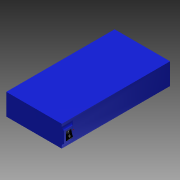
# Autodesk Inventor part: 12 Volt Battery Pack
Saved by Autodesk Inventor 2014 (Build 180170000, 170)
## iProperties
Created: 2014-02-26
Part Number: 12 Volt Battery Pack
Material: Generic
Document SubType Name: Modeling
Designer: Spooner
Density: 1 g/cm^3
Appearance: Blue - Wall Paint - Glossy
Author: Spooner
Autodesk Inventor part; units mm, degrees
ref_plane "YZ Plane" through (0, 0, 0) normal (1, 0, 0) x (0, 1, 0)
ref_plane "XZ Plane" through (0, 0, 0) normal (0, 1, 0) x (-1, 0, 0)
ref_plane "XY Plane" through (0, 0, 0) normal (0, 0, 1) x (1, 0, 0)
sketch "Sketch1" plane through (0, 0, 0) normal (0, 1, 0) x (-1, 0, 0)
  line L0 (0, 0) -> (-65.786, 0)
  line L1 (-65.786, 0) -> (-65.786, -128.524)
  line L2 (-65.786, -128.524) -> (0, -128.524)
  line L3 (0, -128.524) -> (0, 0)
  dimension "d0" = 128.524
  dimension "d1" = 65.786
  constraints: 8 end point, 2 parallel, 1 horizontal, 1 perpendicular
  measures "d0" distance of L2.end L0.start
  measures "d1" distance of L0.start L0.end
extrude "Extrusion1" add sketch "Sketch1" along normal blind 25.4
sketch "Sketch2" plane through (0, 0, -128.524) normal (-1, 0, 0) x (0, 0, 1)
  line L0 (0, 0) -> (128.524, 0) projected
  line L1 (128.524, 0) -> (128.524, 25.4) projected
  line L2 (0, 25.4) -> (128.524, 25.4) projected
  circle A0 centre (126.111, 14.351) radius 1.651
  circle A1 centre (126.111, 11.049) radius 1.651
  point P0 (128.524, 12.7)
  dimension "d4" = 3.302
  dimension "d5" = 11.049
  dimension "d6" = 11.049
  dimension "d7" = 0.762
  constraints: 2 centre point, 2 equal radius, 1 midpoint, 1 vertical alignment
  measures "d4" diameter of A1
  measures "d5" distance from line of L2 A0.centre
  measures "d6" distance from line of L0 A1.centre
  measures "d7" distance edge to line of A0 L1
extrude "Extrusion2" cut sketch "Sketch2" against normal blind 0.762
sketch "Sketch3" plane through (65.786, 0, 0) normal (1, 0, 0) x (0, 0, -1)
  line L0 (0, 0) -> (128.524, 0) projected
  line L1 (0, 25.4) -> (128.524, 25.4) projected
  line L2 (0, 0) -> (0, 25.4) projected
  line L3 (0, 19.812) -> (10.414, 19.812)
  line L4 (10.414, 19.812) -> (10.414, 5.588)
  line L5 (10.414, 5.588) -> (0, 5.588)
  line L6 (0, 5.588) -> (0, 19.812)
  dimension "d10" = 14.224
  dimension "d11" = 10.414
  dimension "d12" = 5.588
  dimension "d13" = 5.588
  constraints: 8 end point, 2 parallel, 1 horizontal, 1 perpendicular, 1 point on line
  measures "d10" distance of L3.end L4.end
  measures "d11" distance of L3.start L3.end
  measures "d12" distance between parallel lines of L1 L3
  measures "d13" distance between parallel lines of L0 L5
extrude "Extrusion3" add sketch "Sketch3" along normal blind 2.54
fillet "Fillet1" radius 3.175 3 edges at (65.786, 19.812, -5.207) (65.786, 12.7, -10.414) (65.786, 5.588, -5.207)
sketch "Sketch4" plane through (68.326, 0, 0) normal (1, 0, 0) x (0, 0, -1)
  line L0 (0, 19.812) -> (0, 5.588) projected
  circle A0 centre (13.5249, 12.7) radius 0.635
  line L1 (13.5249, 2.4771) -> (13.5249, 22.9229) projected
  line L2 (0, 19.812) -> (0, 5.588) projected
  line L3 (0, 5.588) -> (10.414, 5.588) projected
  line L4 (10.414, 5.588) -> (10.414, 19.812) projected
  line L5 (10.414, 19.812) -> (0, 19.812) projected
  point P0 (0, 0)
  point P1 (0, 12.7)
  point P2 (13.5249, 12.7)
  dimension "d17" = 1.27
  constraints: 2 midpoint, 1 centre point, 1 coincident, 1 horizontal alignment
  measures "d17" diameter of A0
extrude "Extrusion4" cut sketch "Sketch4" against normal blind 2.667 contours A0 L1 | L1 A0
ref_plane "Work Plane1" through (0, 0, -2.54) normal (0, 0, 1) x (1, 0, 0)
sketch "Sketch5" plane through (0, 0, -2.54) normal (0, 0, 1) x (1, 0, 0)
  line L0 (68.326, 19.812) -> (68.326, 5.588) projected
  line L1 (68.326, 17.526) -> (68.326, 7.874)
  arc A0 (68.326, 17.526) -> (70.104, 9.906) centre (85.5436, 17.526) ccw
  arc A1 (68.326, 7.874) -> (70.104, 9.906) centre (68.326, 9.6679) ccw
  point P0 (0, 0)
  point P1 (68.326, 12.7)
  point P2 (68.326, 12.7)
  dimension "d21" = 9.652
  dimension "d22" = 7.62
  dimension "d23" = 1.778
  constraints: 4 point on circle, 2 centre point, 2 end point, 2 midpoint, 2 point on line, 1 coincident, 1 line through centre, 1 tangent
  measures "d21" distance of L1.end L1.start
  measures "d22" vertical distance of L1.start A0.end
  measures "d23" horizontal distance of L1.end A0.end
extrude "Extrusion5" add sketch "Sketch5" against normal blind 6.35
ref_plane "Work Plane2" through (68.326, 17.526, -2.54) normal (0.9738412, 0.2272296, 0) x (0, 0, 1)
sketch "Sketch6" plane through (68.326, 17.526, -2.54) normal (0.9738412, 0.2272296, 0) x (0, 0, 1)
  line L0 (0, 7.8247) -> (0, 0) projected
  line L1 (0, 7.8247) -> (0, 0) projected
  line L2 (0, 7.8247) -> (-6.35, 7.8247) projected
  line L3 (-6.35, 0) -> (-6.35, 7.8247) projected
  line L4 (-6.35, 0) -> (0, 0) projected
  line L5 (-3.683, 3.4152) -> (-2.667, 3.4152) construction
  line L6 (-2.667, 3.4152) -> (-2.667, 0.762) construction
  line L7 (-2.667, 0.762) -> (-3.683, 0.762) construction
  line L8 (-3.683, 0.762) -> (-3.683, 3.4152) construction
  line L9 (-4.2799, 7.0627) -> (-2.0701, 7.0627) construction
  line L10 (-2.0701, 7.0627) -> (-2.0701, 4.4177) construction
  line L11 (-2.0701, 4.4177) -> (-4.2799, 4.4177) construction
  line L12 (-4.2799, 4.4177) -> (-4.2799, 7.0627) construction
  spline S0 degree 2 poles (-2.1886, 5.7412) (-2.1886, 5.4119) (-2.2936, 4.9179) (-2.4109, 4.7512) knots 0 0 0 1 2 2 2
  spline S1 degree 2 poles (-2.4109, 4.7512) (-2.5262, 4.5865) (-2.8987, 4.4177) (-3.1663, 4.4177) knots 0 0 0 1 2 2 2
  spline S2 degree 2 poles (-3.1663, 4.4177) (-3.436, 4.4177) (-3.8065, 4.5865) (-3.9238, 4.7553) knots 0 0 0 1 2 2 2
  spline S3 degree 2 poles (-3.9238, 4.7553) (-4.0411, 4.922) (-4.1461, 5.4119) (-4.1461, 5.7412) knots 0 0 0 1 2 2 2
  spline S4 degree 2 poles (-4.1461, 5.7412) (-4.1461, 6.0788) (-4.0411, 6.5563) (-3.9217, 6.7292) knots 0 0 0 1 2 2 2
  spline S5 degree 2 poles (-3.9217, 6.7292) (-3.8024, 6.898) (-3.4257, 7.0627) (-3.1663, 7.0627) knots 0 0 0 1 2 2 2
  spline S6 degree 2 poles (-3.1663, 7.0627) (-2.8926, 7.0627) (-2.5262, 6.8898) (-2.4089, 6.7189) knots 0 0 0 1 2 2 2
  spline S7 degree 2 poles (-2.4089, 6.7189) (-2.2936, 6.5522) (-2.1886, 6.0603) (-2.1886, 5.7412) knots 0 0 0 1 2 2 2
  spline S8 degree 2 poles (-2.8288, 5.7412) (-2.8288, 6.2126) (-2.9831, 6.5934) (-3.1663, 6.5934) knots 0 0 0 1 2 2 2
  spline S9 degree 2 poles (-3.1663, 6.5934) (-3.3495, 6.5934) (-3.506, 6.2126) (-3.506, 5.7392) knots 0 0 0 1 2 2 2
  spline S10 degree 2 poles (-3.506, 5.7392) (-3.506, 5.274) (-3.3495, 4.887) (-3.1663, 4.887) knots 0 0 0 1 2 2 2
  spline S11 degree 2 poles (-3.1663, 4.887) (-2.9852, 4.887) (-2.8288, 5.274) (-2.8288, 5.7412) knots 0 0 0 1 2 2 2
  line L13 (-2.8576, 0.762) -> (-3.4545, 0.762)
  line L14 (-3.4545, 0.762) -> (-3.4545, 3.4152)
  line L15 (-3.4545, 3.4152) -> (-2.8576, 3.4152)
  line L16 (-2.8576, 3.4152) -> (-2.8576, 0.762)
  point P0 (2.54, 1.5419)
  point P1 (-3.175, 7.0627)
  point P2 (-3.175, 3.4152)
  dimension "d26" = 0.762
  dimension "d27" = 0.762
  dimension "d28" = 2.2098
  dimension "d29" = 1.016
  dimension "d30" = 2.0701
  dimension "d31" = 2.0701
  constraints: 2 midpoint, 1 horizontal, 1 vertical alignment, 4 other
  measures "d26" distance between parallel lines of L2 L9
  measures "d27" distance between parallel lines of L4 L7
  measures "d28" distance of L10.end L11.end
  measures "d29" distance of L6.end L7.end
  measures "d30" distance between parallel lines of L3 L12
  measures "d31" distance between parallel lines of L1 L10
emboss "Emboss1" sketch "Sketch6" operation add depth 0.0762 direction (-0.9738412, -0.2272296, 0) contours S0 S1 S2 S3 S4 S5 S6 S7 | L13 L14 L15 L16
equation "\"d5\" = d6"
equation "\"d12\" = d13"
equation "\"d27\" = d26"
equation "\"d30\" = d31"
body "Solid1"
